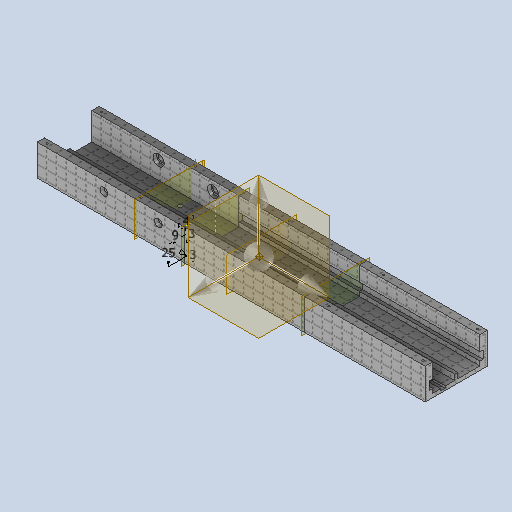
# Autodesk Inventor part: Fuehrungsschiene
Saved by Autodesk Inventor 2024 (Build 280153000, 153)
## iProperties
Created: 2022-04-21
Part Number: Fuehrungsschiene
Material: Generisch
Document SubType Name: Modeling
Designer: 123St
Density: 0.699137 g/cm^3
Appearance: Gehont
Mass: 355.65 g
Surface Area: 1786.68 cm^2
Volume: 508.698 cm^3
GuidanceTrack_Length: 500,000 mm
GuidanceTrac_Width: 80,000 mm
TopLit_Fixhole_Edge_Dist: 8,000 mm
Author: 123St
Autodesk Inventor part; units mm, degrees
sketch "Skizze1" plane through (0, 0, 0) normal (1, 0, 0) x (0, 1, 0)
  line L0 (9, -2) -> (9, 2)
  line L1 (9, 2) -> (2, 2)
  line L2 (2, 2) -> (2, 30)
  line L3 (2, 30) -> (7.5, 30)
  line L4 (7.5, 30) -> (7.5, 34.5)
  line L5 (7.5, 34.5) -> (18, 34.5)
  line L6 (18, 34.5) -> (18, 30)
  line L7 (18, 30) -> (20, 30)
  line L8 (20, 30) -> (20, 40)
  line L9 (20, 40) -> (0, 40)
  line L10 (0, 40) -> (0, -40)
  line L11 (0, -40) -> (20, -40)
  line L12 (20, -40) -> (20, -30)
  line L13 (20, -30) -> (18, -30)
  line L14 (18, -30) -> (18, -34.5)
  line L15 (18, -34.5) -> (7.5, -34.5)
  line L16 (7.5, -34.5) -> (7.5, -30)
  line L17 (2, -30) -> (2, -2)
  line L18 (2, -2) -> (9, -2)
  line L19 (7.5, -30) -> (2, -30)
  line L20 (20, 40) -> (37, 40)
  line L21 (37, 40) -> (37, 30)
  line L22 (37, 30) -> (20, 30)
  line L23 (20, -30) -> (37, -30)
  line L24 (37, -30) -> (37, -40)
  line L25 (37, -40) -> (20, -40)
  line L26 (0, 40) -> (-3, 40)
  line L27 (-3, 40) -> (-3, -40)
  line L28 (-3, -40) -> (0, -40)
  line L29 (0, -40) -> (0, 40)
  point P0 (0, 0)
  dimension "d0" = 4
  dimension "d2" = 2
  dimension "d3" = 7
  dimension "d4" = 28
  dimension "d5" = 28
  dimension "d7" = 10.5
  dimension "d8" = 10.5
  dimension "d9" = 2
  dimension "d10" = 20
  dimension "d13" = 2
  dimension "d15" = 4.5
  dimension "d16" = 4.5
  dimension "d18" = 17
  dimension "GuidanceTrac_Width" = 80
  dimension "d41" = 3
  dimension "d75" = 10
  dimension "d76" = 10
  constraints: 60 end point, 18 perpendicular, 11 point on line, 5 parallel, 2 horizontal, 1 collinear, 1 midpoint, 1 vertical
  measures "d0" distance of L0.start L0.end
  measures "d2" distance from line of point (0, 0) L1
  measures "d3" distance of L0.end L1.end
  measures "d4" distance between parallel lines of L18 L19
  measures "d5" distance between parallel lines of L1 L3
  measures "d7" distance of L4.end L5.end
  measures "d8" distance of L14.end L15.end
  measures "d9" distance of L6.end L7.end
  measures "d10" distance between parallel lines of L12 L10
  measures "d13" distance between parallel lines of L10 L17
  measures "d15" distance of L3.end L4.end
  measures "d16" distance of L15.end L16.end
  measures "d18" distance between parallel lines of L21 L8
  measures "GuidanceTrac_Width" distance between parallel lines of L11 L9
  measures "d41" distance between parallel lines of L10 L27
  measures "d75" distance between parallel lines of L22 L20
  measures "d76" distance between parallel lines of L25 L23
extrude "Extrusion1" add sketch "Skizze1" along normal blind 500 contours L18 L17 L19 L16 L15 L14 L13 L12 L11 L10 L9 L8 L7 L6 L5 L4 L3 L2 L1 L0 | L23 L24 L25 L12 | L8 L20 L21 L22
ref_plane "Arbeitsebene1" through (0, 0, 0) normal (0, 0, 1) x (1, 0, 0)
ref_plane "Arbeitsebene3" through (0, 2, 20.2) normal (0, 0, 1) x (1, 0, 0)
ref_plane "Arbeitsebene2" through (0, 2, 14.2) normal (0, 0, 1) x (1, 0, 0)
sketch "Skizze2" plane through (0, 2, 30) normal (0, 1, 0) x (1, 0, 0)
  line L0 (0, 9.8) -> (500, 9.8)
  line L1 (500, 9.8) -> (500, 15.8)
  line L2 (500, 15.8) -> (0, 15.8)
  line L3 (0, 15.8) -> (0, 9.8)
  line L4 (600, 30) -> (-100, 30) construction
  line L5 (500, 28) -> (500, 0) construction
  line L6 (0, 28) -> (0, 0) construction
  line L7 (0, 12.8) -> (500, 12.8) construction
  dimension "d73" = 6
  dimension "d74" = 17.2
  constraints: 10 end point, 2 collinear, 2 horizontal, 2 midpoint, 2 parallel, 2 point on line, 1 perpendicular
  measures "d73" distance between parallel lines of L2 L0
  measures "d74" distance between parallel lines of L4 L7
extrude "Extrusion2" cut sketch "Skizze2" against normal blind 3
sketch "Skizze3" plane through (0, 37, 40) normal (0, 1, 0) x (1, 0, 0)
  line L0 (0, 10) -> (0, 0) construction
  line L1 (0, 0) -> (500, 0) construction
  line L2 (500, 10) -> (500, 0) construction
  line L3 (0, 10) -> (500, 10) construction
  line L4 (500, 0) -> (500, 80) construction
  line L5 (500, 5) -> (0, 5) construction
  line L6 (0, 0) -> (0, 80) construction
  line L7 (600, 40) -> (-100, 40) construction
  line L8 (0, 70) -> (0, 80) construction
  line L9 (0, 80) -> (500, 80) construction
  line L10 (500, 70) -> (500, 80) construction
  line L11 (0, 70) -> (500, 70) construction
  line L12 (500, 75) -> (0, 75) construction
  line L13 (0, 75) -> (500, 75) construction
  point P0 (0, 40)
  point P1 (492, 5)
  point P2 (371, 5)
  point P3 (250, 5)
  point P4 (129, 5)
  point P5 (8, 5)
  point P6 (492, 75)
  point P7 (371, 75)
  point P8 (250, 75)
  point P9 (129, 75)
  point P10 (8, 75)
  dimension "TopLit_Fixhole_Edge_Dist" = 8
  dimension "d26" = 500
  dimension "d29" = 121
  dimension "d77" = 10
  dimension "d78" = 5
  constraints: 14 end point, 9 symmetric about line, 3 point on line, 1 horizontal, 1 perpendicular, 4 other
  measures "TopLit_Fixhole_Edge_Dist" distance from line of L2 point (492, 5)
  measures "d26" distance between parallel lines of L0 L2
  measures "d29" distance of point (492, 5) point (371, 5)
  measures "d77" distance between parallel lines of L3 L1
  measures "d78" distance between parallel lines of L1 L5
hole "Bohrung1" at (492, 37, 35) at (371, 37, 35) at (250, 37, 35) at (129, 37, 35) at (8, 37, 35) at (8, 37, -35) at (129, 37, -35) at (250, 37, -35) at (371, 37, -35) at (492, 37, -35) direction (0, -1, 0) diameter 2.459 depth 8 tip angle 118 thread size "M3x0.5" class "6H" standard "ISO Metric profile"
extrude "Extrusion3" add sketch "Skizze1" along normal up to surface (500 mm away) contours L28 L27 L26 L10
ref_plane "Arbeitsebene5" through (0, 17, 40) normal (0, 1, 0) x (1, 0, 0)
mirror "Spiegeln1" about plane through (0, 17, 40) normal (0, 1, 0) of "Bohrung1"
ref_plane "Arbeitsebene6" through (8, 37, 35) normal (-1, 0, 0) x (0, -1, 0)
ref_plane "Arbeitsebene7" through (129, 33, 35) normal (-1, 0, 0) x (0, 1, 0)
sketch "Skizze4" plane through (0, 37, 40) normal (0, 0, 1) x (1, 0, 0)
  line L0 (8, 7.4) -> (8, -44.4) construction
  line L1 (129, -44.4) -> (129, 7.4) construction
  line L2 (0, -19) -> (0, 0) construction
  line L3 (0, 0) -> (500, 0) construction
  line L4 (500, -19) -> (500, 0) construction
  line L5 (0, -19) -> (500, -19) construction
  circle A0 centre (86, -12.25) radius 5
  circle A1 centre (156, -12.25) radius 5
  line L6 (86, -12.25) -> (156, -12.25) construction
  point P0 (0, -37)
  point P1 (0, -9.5)
  point P2 (121, -12.25)
  dimension "d46" = 10
  dimension "d47" = 10
  dimension "d48" = 70
  dimension "d49" = 113
  dimension "d101" = 6.75
  constraints: 2 centre point, 2 end point, 2 midpoint
  measures "d46" diameter of A0
  measures "d47" diameter of A1
  measures "d48" distance of L6.end L6.start
  measures "d49" distance from line of L0 point (121, -12.25)
  measures "d101" distance between parallel lines of L6 L5
extrude "Extrusion4" cut sketch "Skizze4" against normal through all
ref_plane "Arbeitsebene8" through (95, 0, 0) normal (-1, 0, 0) x (0, 0, 1)
sketch "Skizze5" plane through (0, 0, 0) normal (-1, 0, 0) x (0, 0, 1)
  line L0 (2, 2) -> (14.2, 2) projected
  line L1 (2, 9) -> (2, 2) projected
  line L2 (-2, 9) -> (2, 9) projected
  line L3 (-2, 2) -> (-2, 9) projected
  line L4 (-30, 2) -> (-2, 2) projected
  line L5 (-30, 7.5) -> (-30, 2) projected
  line L6 (-34.5, 7.5) -> (-30, 7.5) projected
  line L7 (-34.5, 18) -> (-34.5, 7.5) projected
  line L8 (-30, 18) -> (-34.5, 18) projected
  line L9 (-30, 37) -> (-30, 18) projected
  line L10 (-40, 37) -> (-30, 37) projected
  line L11 (-40, -3) -> (-40, 37) projected
  line L12 (40, -3) -> (-40, -3) projected
  line L13 (40, 37) -> (40, -3) projected
  line L14 (30, 37) -> (40, 37) projected
  line L15 (30, 18) -> (30, 37) projected
  line L16 (34.5, 18) -> (30, 18) projected
  line L17 (34.5, 7.5) -> (34.5, 18) projected
  line L18 (30, 7.5) -> (34.5, 7.5) projected
  line L19 (30, 2) -> (30, 7.5) projected
  line L20 (-30, 18) -> (-34.5, 18) projected
  line L21 (-34.5, 7.5) -> (-30, 7.5) projected
  line L22 (-34.5, 18) -> (-30, 18)
  line L23 (-30, 18) -> (-30, 7.5)
  line L24 (-30, 7.5) -> (-34.5, 7.5)
  line L25 (-34.5, 7.5) -> (-34.5, 18)
  line L26 (20.2, 0) -> (14.2, 0)
  line L27 (14.2, 0) -> (14.2, 2)
  line L28 (14.2, 2) -> (20.2, 2)
  line L29 (-2, 2) -> (-2, 9) projected
  line L30 (2, 2) -> (14.2, 2) projected
  line L31 (-2, 9) -> (2, 9)
  line L32 (2, 9) -> (2, 2)
  line L33 (2, 2) -> (-2, 2)
  line L34 (-2, 2) -> (-2, 9)
  line L35 (34.5, 7.5) -> (34.5, 18) projected
  line L36 (30, 2) -> (30, 7.5) projected
  line L37 (34.5, 18) -> (30, 18)
  line L38 (30, 18) -> (30, 7.5)
  line L39 (30, 7.5) -> (34.5, 7.5)
  line L40 (34.5, 7.5) -> (34.5, 18)
  line L41 (-40, 37) -> (-30, 37) projected
  line L42 (-30, 7.5) -> (-30, 2) projected
  line L43 (-32, 37) -> (-30, 37)
  line L44 (-30, 37) -> (-30, 2)
  line L45 (-30, 2) -> (-32, 2)
  line L46 (-32, 2) -> (-32, 37)
  line L47 (30, 37) -> (40, 37) projected
  line L48 (32, 37) -> (30, 37)
  line L49 (30, 37) -> (30, 2)
  line L50 (30, 2) -> (32, 2)
  line L51 (32, 2) -> (32, 37)
  line L52 (20.2, 2) -> (20.2, 0) projected
  line L53 (14.2, 0) -> (20.2, 0) projected
  line L54 (14.2, 0) -> (14.2, 2) projected
  line L55 (20.2, 2) -> (30, 2) projected
  line L56 (20.2, 0) -> (20.2, 2)
  line L57 (14.2, 0) -> (20.2, 0) projected
  line L58 (20.2, 2) -> (30, 2) projected
  point P0 (0, 0)
  point P1 (-2, 2)
  point P2 (20.2, 2)
  dimension "d52" = 8
  dimension "d53" = 8
  constraints: 48 end point, 12 equal length, 6 horizontal, 6 perpendicular, 4 collinear, 2 point on line, 1 vertical
  measures "d52" distance between parallel lines of L13 L51
  measures "d53" distance between parallel lines of L46 L11
extrude "Extrusion5" add sketch "Skizze5" against normal blind 189.5 contours L28 L52 L26 L27 | L6 L46 L8 L23 | L38 L16 L51 L18 | L6 L7 L8 L46 | L51 L16 L17 L18
ref_plane "Arbeitsebene14" through (189.5, 15.375, -34.5) normal (-1, 0, 0) x (0, -1, 0)
thicken "Verdickung1" operation add thickness 0.5 both sides no extend neighbours yes toward (0, -1, 0) faces at (396.5, 0, 16.2)
ref_plane "Arbeitsebene12" through (129, 33, -35) normal (1, 0, 0) x (0, 1, 0)
ref_plane "Arbeitsebene9" through (250, 33, -35) normal (1, 0, 0) x (0, 1, 0)
ref_plane "Arbeitsebene11" through (310.5, 33, -35) normal (1, 0, 0) x (0, 1, 0)
ref_plane "Arbeitsebene10" through (371, 33, -35) normal (1, 0, 0) x (0, 1, 0)
ref_plane "Arbeitsebene13" through (189.5, 33, -35) normal (1, 0, 0) x (0, 1, 0)
sketch "Skizze8" plane through (0, 0, 0) normal (0, 0, 1) x (1, 0, 0)
  circle A0 centre (86, 24.75) radius 5 construction
  circle A1 centre (86, 24.75) radius 7.1
  circle A2 centre (156, 24.75) radius 7.1
  arc A3 (151, 24.75) -> (151, 24.75) centre (156, 24.75) ccw construction
  point P0 (0, 0)
  dimension "d69" = 14.2
  dimension "d70" = 14.2
  constraints: 3 coincident, 2 centre point
  measures "d69" diameter of A1
  measures "d70" diameter of A2
extrude "Extrusion9" cut sketch "Skizze8" along normal mid plane 70
thicken "Verdickung2" operation add thickness 0.5 both sides no extend neighbours yes toward (0, 0, 1) faces at (396.5, 24.3333, 30)
thicken "Verdickung3" operation add thickness 0.5 both sides no extend neighbours yes toward (0, 0, -1) faces at (396.5, 24.3333, -30)
sketch "Skizze9" plane through (0, -3, -40) normal (0, -1, 0) x (1, 0, 0)
  line L0 (189.5, 60.2) -> (500, 60.2) construction
  line L1 (500, 60.2) -> (500, 54.2) construction
  line L2 (500, 54.2) -> (189.5, 54.2) construction
  line L3 (500, 57.2) -> (189.5, 57.2) construction
  line L4 (189.5, 54.2) -> (189.5, 60.2) construction
  line L5 (189.5, 54.2) -> (189.5, 60.2) projected
  point P0 (0, 40)
  point P1 (474.8673, 57.2)
  point P2 (423.9733, 57.2)
  point P3 (373.0793, 57.2)
  point P4 (322.1853, 57.2)
  point P5 (271.2913, 57.2)
  point P6 (220.3973, 57.2)
  dimension "d83" = 25.1327
  dimension "d84" = 310.5
  dimension "d87" = 50.894
  constraints: 4 end point, 3 midpoint, 1 collinear, 1 horizontal, 1 point on line, 5 other
  measures "d83" distance from line of L1 point (474.867, 57.2)
  measures "d84" distance of L3.end L3.start
  measures "d87" distance of point (474.867, 57.2) point (423.973, 57.2)
hole "Bohrung2" at (474.8673, -3, 17.2) at (423.9733, -3, 17.2) at (373.0793, -3, 17.2) at (322.1853, -3, 17.2) at (271.2913, -3, 17.2) at (220.3973, -3, 17.2) direction (0, 1, 0) diameter 3.4 depth 5.5 countersink diameter 7.5 countersink angle 90 clearance for "Innensechskant-Senkkopfschraube DIN EN ISO 10642" size "M3" standard "DIN"
ref_plane "Arbeitsebene15" through (344.75, 15.375, -34.5) normal (-1, 0, 0) x (0, -1, 0)
split body "Trennen1" result two bodies by plane through (189.5, 33, -35) normal (1, 0, 0) first body at (314.0959, -2.5, -18.9125)
split body "Trennen3" result two bodies by plane through (344.75, 15.375, -34.5) normal (-1, 0, 0) bodies 2 first body at (305.471, -2.5, -20.3241)
sketch "Skizze6" plane through (189.5, 0, 0) normal (-1, 0, 0) x (0, 0, 1)
  circle A0 centre (36, 28) radius 1.5
  circle A1 centre (36, 3) radius 1.5
  line L0 (36, 3) -> (36, 28) construction
  line L1 (0, 44.4) -> (0, -7.4) construction
  circle A2 centre (-36, 28) radius 1.5
  circle A3 centre (-36, 3) radius 1.5
  line L2 (-36, 3) -> (-36, 28) construction
  line L3 (40, 37) -> (30.5, 37) construction
  point P0 (0, 0)
  dimension "d61" = 3
  dimension "d62" = 3
  dimension "d63" = 25
  dimension "d99" = 9
  dimension "d100" = 4
  constraints: 4 centre point, 4 end point, 2 symmetric about line, 1 vertical, 2 other
  measures "d61" diameter of A0
  measures "d62" diameter of A1
  measures "d63" distance of L0.start L0.end
  measures "d99" distance from line of L3 L0.end
  measures "d100" distance from line of L3.start L0
extrude "Extrusion7" cut sketch "Skizze6" along normal mid plane 25 bodies 3 4
sketch "Skizze12" plane through (344.75, 15.375, -34.5) normal (-1, 0, 0) x (0, -1, 0)
  circle A0 centre (-12.625, 70.5) radius 1.5 projected
  circle A1 centre (12.375, 70.5) radius 1.5 projected
  circle A2 centre (-12.625, -1.5) radius 1.5 projected
  circle A3 centre (12.375, -1.5) radius 1.5 projected
  point P0 (15.375, 34.5)
extrude "Extrusion10" cut sketch "Skizze12" along normal mid plane 25 bodies 5 4
sketch "Skizze13" plane through (0, 2, -2) normal (0, 1, 0) x (1, 0, 0)
  line L0 (122, 14.25) -> (134.25, 14.25) construction
  arc A0 (122, 17) -> (122, 11.5) centre (122, 14.25) ccw construction
  arc A1 (134.25, 11.5) -> (134.25, 17) centre (134.25, 14.25) ccw construction
  point P0 (0, -2)
  point P1 (128.125, 14.25)
  constraints: 2 end point, 1 horizontal, 1 midpoint
hole "Bohrung3" at (128.125, 2, -16.25) direction (0, -1, 0) diameter 5.5 end through all bodies 3 clearance for "Inbusschraube DIN EN ISO 4762" size "M5" standard "DIN"
equation "\"d2\" = 0.5 * d0"
equation "\"d4\" = d5"
equation "\"d16\" = d15"
equation "\"d78\" = 0.5 * d77"
equation "\"d47\" = d46"
equation "\"d48\" = VerticalDistance"
equation "\"d83\" = 8 * Teilung"
equation "\"Modul\" = 1"
equation "\"Teilung\" = 3.14159 * Modul"
equation "\"VerticalDistance\" = 70"
